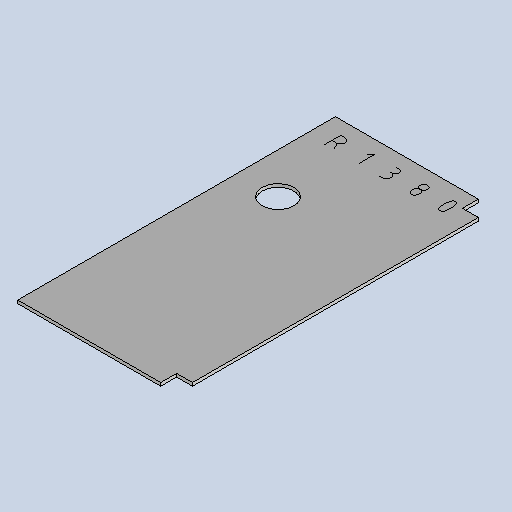
# Autodesk Inventor part: Part13
Saved by Autodesk Inventor 2025.3 (Build 293356030, 356C)
## iProperties
Created: 2026-01-14
Part Number: Part13
Material: Stainless Steel
Document SubType Name: Sheet Metal
Designer: admin
Mass: 311.773 g
Surface Area: 402.973 cm^2
Volume: 38.9717 cm^3
Density: 8 g/cm^3
Sheet Metal Rule: AISI304 2mm Die16
Sheet Metal Width: 100,000 mm
Sheet Metal Length: 200,000 mm
Sheet Metal Area: 20000,000 mm^2
Appearance: Default
Flat Pattern Width: 10 cm
Flat Pattern Length: 20 cm
Flat Pattern Area: 200 cm^2
Author: admin
Autodesk Inventor part; units mm, degrees
ref_plane "YZ Plane" through (0, 0, 0) normal (1, 0, 0) x (0, 1, 0)
ref_plane "XZ Plane" through (0, 0, 0) normal (0, 1, 0) x (-1, 0, 0)
ref_plane "XY Plane" through (0, 0, 0) normal (0, 0, 1) x (1, 0, 0)
sketch "Sketch1" plane through (0, 0, 0) normal (0, 0, 1) x (1, 0, 0)
  line L0 (-50, -100) -> (50, -100)
  line L1 (50, -100) -> (50, 100)
  line L2 (50, 100) -> (-50, 100)
  line L3 (-50, 100) -> (-50, -100)
  line L4 (-50, -100) -> (50, 100) construction
  line L5 (50, -100) -> (-50, 100) construction
  line L6 (50, 100) -> (40, 100)
  line L7 (40, 100) -> (40, 90)
  line L8 (40, 90) -> (50, 90)
  line L9 (50, 90) -> (50, 100)
  line L10 (50, -100) -> (40, -100)
  line L11 (40, -100) -> (40, -90)
  line L12 (40, -90) -> (50, -90)
  line L13 (50, -90) -> (50, -100)
  point P0 (0, 0)
  dimension "d154" = 100
  dimension "d155" = 200
  dimension "d158" = 10
  dimension "d159" = 10
  measures "d154" distance of L1.end L2.end
  measures "d155" distance of L0.end L1.end
  measures "d158" distance of L8.end L7.end
  measures "d159" distance of L7.end L6.end
extrude "Plate5" add sketch "Sketch1" along normal blind 2 contours L3 L2 L7 L8 L1 L12 L11 L0
sketch "Sketch7" plane through (0, 0, 2) normal (0, 0, 1) x (1, 0, 0)
  circle A0 centre (-24.4419, 38.3162) radius 10
  point P0 (0, 0)
  dimension "d157" = 20
  constraints: 1 centre point
  measures "d157" diameter of A0
extrude "Cut1" cut sketch "Sketch7" against normal blind 2
sketch "Sketch8" plane through (0, 0, 2) normal (0, 0, 1) x (1, 0, 0)
  line L0 (-39.1312, 91.8227) -> (16.5981, 91.8227) construction
  line L1 (16.5981, 91.8227) -> (16.5981, 81.3689) construction
  line L2 (16.5981, 81.3689) -> (-39.1312, 81.3689) construction
  line L3 (-39.1312, 81.3689) -> (-39.1312, 91.8227) construction
  point P0 (0, 0)
  constraints: 2 other
mark "Mark2"
body "Solid3"
